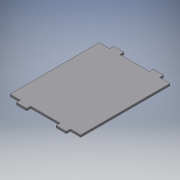
# Autodesk Inventor part: sideWall_R2
Saved by Autodesk Inventor 2017 (Build 210142000, 142)
## iProperties
Created: 2017-06-08
Part Number: sideWall_R2
Material: Generic
Document SubType Name: Modeling
Designer: Paolo
Density: 1 g/cm^3
Appearance: Default
Author: Paolo
Autodesk Inventor part; units mm, degrees
ref_plane "YZ Plane" through (0, 0, 0) normal (1, 0, 0) x (0, 1, 0)
ref_plane "XZ Plane" through (0, 0, 0) normal (0, 1, 0) x (-1, 0, 0)
ref_plane "XY Plane" through (0, 0, 0) normal (0, 0, 1) x (1, 0, 0)
sketch "Sketch1" plane through (0, 0, 0) normal (0, 0, 1) x (1, 0, 0)
  line L0 (15.2, -6) -> (0, -6) projected
  line L1 (15.2, 0) -> (15.2, -6) projected
  line L2 (0, 0) -> (15.2, 0) projected
  line L3 (0, 0) -> (0, -6) projected
  line L4 (73, -6) -> (57.8, -6) projected
  line L5 (73, 0) -> (73, -6) projected
  line L6 (57.8, 0) -> (73, 0) projected
  line L7 (57.8, 0) -> (57.8, -6) projected
  line L8 (57.8, -136) -> (73, -136) projected
  line L9 (57.8, -136) -> (57.8, -151) projected
  line L10 (57.8, -151) -> (73, -151) projected
  line L11 (73, -136) -> (73, -151) projected
  line L12 (0, -136) -> (15.2, -136) projected
  line L13 (0, -136) -> (0, -151) projected
  line L14 (0, -151) -> (15.2, -151) projected
  line L15 (15.2, -136) -> (15.2, -151) projected
  line L16 (0.1, -150.9) -> (0.1, -136.1)
  line L17 (0.1, -136.1) -> (15.1, -136.1)
  line L18 (15.1, -136.1) -> (15.1, -150.9)
  line L19 (15.1, -150.9) -> (0.1, -150.9)
  line L20 (57.9, -150.9) -> (57.9, -136.1)
  line L21 (57.9, -136.1) -> (72.9, -136.1)
  line L22 (72.9, -136.1) -> (72.9, -150.9)
  line L23 (72.9, -150.9) -> (57.9, -150.9)
  line L24 (88, -136) -> (-15, -136) projected
  line L25 (-15, -136) -> (88, -136)
  line L26 (88, -136) -> (88, -6)
  line L27 (88, -6) -> (-15, -6)
  line L28 (-15, -6) -> (-15, -136)
  line L29 (0.1, -5.9) -> (15.1, -5.9)
  line L30 (15.1, -5.9) -> (15.1, -0.1)
  line L31 (15.1, -0.1) -> (0.1, -0.1)
  line L32 (0.1, -0.1) -> (0.1, -5.9)
  line L33 (57.9, -5.9) -> (72.9, -5.9)
  line L34 (72.9, -5.9) -> (72.9, -0.1)
  line L35 (72.9, -0.1) -> (57.9, -0.1)
  line L36 (57.9, -0.1) -> (57.9, -5.9)
  line L37 (72.9, -5.9) -> (72.9, -6)
  line L38 (57.9, -5.9) -> (57.9, -6)
  line L39 (15.1, -5.9) -> (15.1, -6)
  line L40 (0.1, -5.9) -> (0.1, -6)
  line L41 (0.1, -136.1) -> (0.1, -136)
  line L42 (15.1, -136.1) -> (15.1, -136)
  line L43 (57.9, -136.1) -> (57.9, -136)
  line L44 (72.9, -136.1) -> (72.9, -136)
  line L45 (0.1, -141.9) -> (15.1, -141.9)
  line L46 (57.9, -141.9) -> (72.9, -141.9)
  dimension "d0" = 0.1
  dimension "d1" = 0.1
  dimension "d2" = 103
  dimension "d3" = 130
  dimension "d4" = 0.1
  dimension "d5" = 0.1
  dimension "d6" = 5.9
  dimension "d7" = 5.9
  dimension "d8" = 5.9
  constraints: 60 end point, 16 point on line, 7 perpendicular, 2 parallel, 1 horizontal, 12 other
  measures "d0" distance between parallel lines of L13 L16
  measures "d1" distance between parallel lines of L9 L20
  measures "d2" distance of L27.end L26.end
  measures "d3" distance of L26.end L25.end
  measures "d4" distance between parallel lines of L3 L32
  measures "d5" distance between parallel lines of L7 L36
  measures "d6" distance between parallel lines of L24 L45
  measures "d7" distance between parallel lines of L27 L31
  measures "d8" distance between parallel lines of L24 L46
extrude "Extrusion1" add sketch "Sketch1" along normal blind 3 contours L27 L4 L26 L24 L8 L12 L28 L0 | L0 L40 L29 L39 | L29 L32 L31 L30 | L38 L33 L37 L4 | L36 L35 L34 L33 | L12 L42 L17 L41 | L17 L18 L45 L16 | L44 L21 L43 L8 | L22 L46 L20 L21
equation "\"d6\" = d7"
equation "\"d8\" = d7"
body "Solid1"
